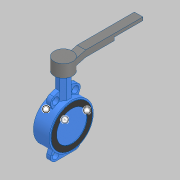
# Autodesk Inventor part: BUTTERFLY VALVE MANUAL WAFER TYPE DN100
Saved by Autodesk Inventor 2017 (Build 210142000, 142)
## iProperties
Created: 2017-11-22
Part Number: BUTTERFLY VALVE MANUAL WAFER TYPE DN100
Material: GG25
Document SubType Name: Modeling
Designer: Demarec
Density: 7.85 g/cm^3
Appearance: Steel - Cast(1)
Description: BELVEN BV10
Catalog Web Link: http://www.pocketbrewery.com
Author: Demarec
Autodesk Inventor part; units mm, degrees
ref_plane "YZ Plane" through (0, 0, 0) normal (1, 0, 0) x (0, 1, 0)
ref_plane "XZ Plane" through (0, 0, 0) normal (0, 1, 0) x (-1, 0, 0)
ref_plane "XY Plane" through (0, 0, 0) normal (0, 0, 1) x (1, 0, 0)
sketch "Sketch1" plane through (0, 0, 0) normal (0, 1, 0) x (-1, 0, 0)
  circle A0 centre (0, 0) radius 72.5
  circle A1 centre (0, 0) radius 77.5
  circle A2 centre (0, 0) radius 53.5
  circle A3 centre (0, 0) radius 90 construction
  line L0 (0, 0) -> (-34.4415, 83.1492) construction
  circle A4 centre (-34.4415, 83.1492) radius 12
  line L1 (0, 154) -> (-32.5, 154)
  line L2 (-32.5, 154) -> (-32.5, 198)
  line L3 (-32.5, 198) -> (0, 198)
  line L4 (0, 198) -> (0, 154)
  line L5 (0, 140.825) -> (0, 198)
  line L6 (20, 74.8749) -> (-20, 74.8749)
  line L7 (-20, 74.8749) -> (-20, 154)
  line L8 (-20, 154) -> (20, 154)
  line L9 (20, 154) -> (20, 74.8749)
  line L10 (0, 0) -> (0, 198)
  line L11 (265, 193) -> (63.4449, 193)
  line L12 (63.4449, 193) -> (63.4449, 171)
  line L13 (63.4449, 171) -> (265, 171)
  line L14 (265, 171) -> (265, 193)
  line L15 (63.4449, 193) -> (0, 176)
  line L16 (63.4449, 171) -> (0, 154)
  line L17 (0, 154) -> (0, 176)
  arc A5 (-20, 106.132) -> (-41.3298, 99.779) centre (0, 0) ccw
  arc A6 (-41.3298, 99.779) -> (-51.0713, 76.2609) centre (-34.4415, 83.1492) ccw
  line L18 (-51.0713, 76.2609) -> (-45.4768, 62.7544)
  line L19 (-45.4768, 62.7544) -> (-20, 74.8749)
  line L20 (-20, 74.8749) -> (-20, 106.132)
  circle A7 centre (-34.4415, -83.1492) radius 12
  line L21 (0, 0) -> (-34.4415, -83.1492) construction
  line L22 (-45.4768, -62.7544) -> (-51.0713, -76.2609)
  arc A8 (-51.0713, -76.2609) -> (-34.4415, -101.1492) centre (-34.4415, -83.1492) ccw
  line L23 (-34.4415, -101.1492) -> (0, -101.1492)
  line L24 (0, -101.1492) -> (0, -77.5)
  line L25 (0, -77.5) -> (-45.4768, -62.7544)
  line L26 (265, 182) -> (164.2224, 182)
  line L27 (164.2224, 182) -> (164.2224, 171)
  line L28 (164.2224, 171) -> (265, 171)
  line L29 (265, 171) -> (265, 182)
  dimension "oDiaGasket" = 145
  dimension "oDiaOutside" = 155
  dimension "oDiaInside" = 107
  dimension "oHoledia" = 24
  dimension "oStemThick" = 40
  dimension "oAngleFirstBolt" = 22.5
  dimension "oKcircle" = 180
  dimension "oDiaTop" = 65
  dimension "oHeightTop" = 44
  dimension "oHandleLenght" = 265
  dimension "d10" = 5
  dimension "d11" = 15
  dimension "d13" = 6
  dimension "oCenterTop" = 198
  dimension "d32" = 22.5
  dimension "d33" = 6
  constraints: 60 end point, 13 point on circle, 11 parallel, 9 centre point, 5 perpendicular, 4 coincident, 4 horizontal, 4 midpoint, 4 point on line, 4 tangent, 3 collinear, 3 concentric, 1 equal radius, 1 vertical
  measures "oDiaGasket" diameter of A0
  measures "oDiaOutside" diameter of A1
  measures "oDiaInside" diameter of A2
  measures "oHoledia" diameter of A4
  measures "oStemThick" distance between parallel lines of L9 L7
  measures "oAngleFirstBolt" angle of L0 L7
  measures "oKcircle" diameter of A3
  measures "oDiaTop" diameter of L2 L10
  measures "oHeightTop" distance of L1.end L2.end
  measures "oHandleLenght" distance from line of L3.end L14
  measures "d10" distance between parallel lines of L11 L3
  measures "d11" angle of L15 L11
  measures "d13" radial gap between concentric circles of A6 A4
  measures "oCenterTop" distance from line of L3 point (0, 0)
  measures "d32" angle of L10 L21
  measures "d33" radial gap between concentric circles of A8 A7
sketch "Sketch2" plane through (0, 0, 0) normal (0, 1, 0) x (-1, 0, 0)
  circle A0 centre (0, 0) radius 77.5 projected
  circle A1 centre (0, 0) radius 72.5 projected
  circle A2 centre (0, 0) radius 53.5 projected
extrude "Extrusion4" add sketch "Sketch2" along normal mid plane 56 contours A0 | A1 | A2
extrude "Extrusion5" add sketch "Sketch2" along normal mid plane 60 contours A1
extrude "Extrusion6" add sketch "Sketch1" along normal mid plane 40 contours A1 L10 L5 L8 L9 | L7 L1 L5 L10 A1
revolve "Revolution1" add sketch "Sketch1" angle 360 about axis through (0, 0, 0) along (0, 0, 1) contours L1 L2 L3 L4
extrude "Extrusion8" add sketch "Sketch1" along normal mid plane 15 contours A2 | A1 L18 A6 A5 L7 | L24 L23 A8 L22 A1
mirror "Mirror1" about plane through (0, 0, 0) normal (1, 0, 0) of "Extrusion8"
extrude "Extrusion9" add sketch "Sketch1" along normal mid plane 30 contours L4 L15 L12 L16 | L12 L11 L14 L26 L27 L13
chamfer "Chamfer1" distance 12 angle 45 4 edges at (-20, 20, 114.4374) (20, 20, 114.4374) (-20, -20, 114.4374) (20, -20, 114.4374)
equation "\"d32\" = oAngleFirstBolt"
equation "\"d33\" = d13"
equation "\"d25\" = oStemThick"
body "Solid2"
